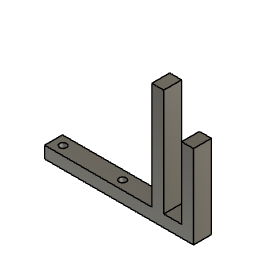
sensor_mod_handle v9 (Autodesk Fusion 360 design; units mm, degrees)
Autodesk Fusion 360 part; units mm, degrees
sketch "Sketch1" plane through (0, 0, 0) normal (0, 0, 1) x (1, 0, 0)
  line L0 (60, 10) -> (70, 10)
  line L1 (70, 10) -> (70, -90)
  line L2 (70, -90) -> (60, -90)
  line L3 (60, -90) -> (60, 10)
  line L4 (70, 10) -> (85, 10)
  line L5 (85, 10) -> (85, 0)
  line L6 (85, 0) -> (70, 0)
  line L7 (70, 0) -> (70, 10)
  line L8 (60, 0) -> (-30, 0)
  line L9 (-30, 0) -> (-30, 10)
  line L10 (-30, 10) -> (60, 10)
  line L11 (60, 10) -> (60, 0)
  line L12 (85, 10) -> (95, 10)
  line L13 (95, 10) -> (95, -60)
  line L14 (95, -60) -> (85, -60)
  line L15 (85, -60) -> (85, 10)
  dimension "d3" = 10
  dimension "d4" = 100
  dimension "d5" = 15
  dimension "d8" = 90
  dimension "d21" = 10
  dimension "d22" = 70
  constraint horizontal L0
  constraint vertical L1
  constraint horizontal L2
  constraint vertical L3
  constraint horizontal L4
  constraint vertical L5
  constraint horizontal L6
  constraint vertical L7
  constraint horizontal L8
  constraint vertical L9
  constraint horizontal L10
  constraint vertical L11
  constraint coincident L3 L8.start
  constraint horizontal L12
  constraint vertical L13
  constraint horizontal L14
  constraint vertical L15
  measures "d3" distance of L0.start L0.end
  measures "d4" distance of L0.end L1.end
  measures "d5" distance of L5.end L6.end
  measures "d8" distance of L9.end L0.start
  measures "d21" distance of L4.end L12.end
  measures "d22" distance of L4.end L14.end
extrude "Extrude1" add sketch "Sketch1" along normal blind 10
extrude "Extrude2" add 1 faces at (91.6667, -16.6667, 10) along direction (0, 0, 1) blind 5
sketch "Sketch3" plane through (0, 0, 0) normal (0, -1, 0) x (1, 0, 0)
  line L0 (-30, 0) -> (60, 0)
  line L1 (60, 0) -> (60, 15)
  line L2 (60, 15) -> (-30, 15)
  line L3 (-30, 15) -> (-30, 0)
  line L4 (-30, 15) -> (-27, 15)
  line L5 (-27, 15) -> (-27, 0)
  line L6 (-27, 0) -> (-30, 0)
  line L7 (-30, 0) -> (-30, 15)
  line L8 (-27, 15) -> (-17, 15)
  line L9 (-17, 15) -> (-17, 0)
  line L10 (-17, 0) -> (-27, 0)
  line L11 (-27, 0) -> (-27, 15)
  circle A0 centre (-22, 7.5) radius 1.5
  line L12 (23, 15) -> (33, 15)
  line L13 (33, 15) -> (33, 0)
  line L14 (33, 0) -> (23, 0)
  line L15 (23, 0) -> (23, 15)
  circle A1 centre (28, 7.5) radius 1.5
  dimension "d13" = 3
  dimension "d14" = 10
  dimension "d15" = 3
  dimension "d16" = 10
  dimension "d17" = 40
  dimension "d18" = 3
  constraint horizontal L4
  constraint vertical L5
  constraint horizontal L6
  constraint vertical L7
  constraint coincident L2.end L3.start
  constraint horizontal L8
  constraint vertical L9
  constraint horizontal L10
  constraint vertical L11
  constraint horizontal L12
  constraint vertical L13
  constraint horizontal L14
  constraint vertical L15
  constraint coincident L0 L13.end
  constraint coincident L2 L12.start
  measures "d13" distance of L2.end L4.end
  measures "d14" distance of L4.end L8.end
  measures "d15" diameter of A0
  measures "d16" distance of L12.start L12.end
  measures "d17" distance of L9 L15
  measures "d18" diameter of A1
extrude "Extrude3" cut sketch "Sketch3" against normal blind 30 contours A0 | A1
sketch "Sketch4" plane through (0, 0, 0) normal (0, -1, 0) x (1, 0, 0)
  circle A0 centre (-22, 7.5) radius 1.5
  circle A1 centre (28, 7.5) radius 1.5
  line L0 (-30, 0) -> (60, 0)
  line L1 (60, 0) -> (60, 15)
  line L2 (60, 15) -> (-30, 15)
  line L3 (-30, 15) -> (-30, 0)
  circle A2 centre (28, 7.5) radius 3
  circle A3 centre (-22, 7.5) radius 3
  dimension "d23" = 6
  dimension "d24" = 6
  constraint concentric A1 A2
  constraint concentric A0 A3
  measures "d23" diameter of A2
  measures "d24" diameter of A3
extrude "Extrude4" cut sketch "Sketch4" against normal blind 7 contours A2 | A3
move_body "Move1" bodies 1 to x (1, 0, 0) y (0, 0, -1) z (0, 1, 0) at (0, 0, 0)
move_body "Move2" bodies 1 to x (1, 0, 0) y (0, 1, 0) z (0, 0, 1) at (0, 0, 10)
